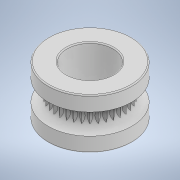
# Autodesk Inventor part: ToothedLoadedWheel_10mm
Saved by Autodesk Inventor 2021 (Build 250183000, 183)
## iProperties
Created: 2021-07-08
Part Number: ToothedLoadedWheel_10mm
Material: Generic
Document SubType Name: Modeling
Designer: zmac845
Density: 1 g/cm^3
Appearance: Default
Author: zmac845
Autodesk Inventor part; units mm, degrees
ref_plane "YZ Plane" through (0, 0, 0) normal (1, 0, 0) x (0, 1, 0)
ref_plane "XZ Plane" through (0, 0, 0) normal (0, 1, 0) x (-1, 0, 0)
ref_plane "XY Plane" through (0, 0, 0) normal (0, 0, 1) x (1, 0, 0)
sketch "Sketch1" plane through (0, 0, 0) normal (0, 0, 1) x (1, 0, 0)
  line L0 (0, 0) -> (20, 0)
  line L1 (20, 0) -> (20, 12)
  line L2 (20, 12) -> (0, 12)
  line L3 (0, 12) -> (0, 0)
  line L4 (0, 0) -> (11, 0)
  line L5 (11, 0) -> (11, 12)
  line L6 (11, 12) -> (0, 12)
  line L7 (0, 12) -> (0, 0)
  line L8 (20, 12) -> (20, 12)
  arc A0 (15, 12) -> (23.1054, 8.0813) centre (20, 12) ccw
  point P0 (20, 7)
  dimension "d0" = 20
  dimension "d1" = 12
  dimension "d2" = 11
  dimension "d3" = 0
  dimension "d4" = 5
  constraints: 18 end point, 4 parallel, 3 perpendicular, 2 horizontal, 2 point on circle, 2 point on line, 1 centre point, 1 coincident
  measures "d0" distance of L2.end L1.end
  measures "d1" distance of L1.end L0.end
  measures "d2" distance of L6.end L5.end
  measures "d3" distance of L1.end L8.end
  measures "d4" radius of A0
revolve "Revolution1" add sketch "Sketch1" angle 360 about axis through (0, 12, 0) along (0, -1, 0) contours L5 L2 A0 L1 L0
mirror "Mirror1" about plane through (15, 12, 0) normal (0, 1, 0) of "Revolution1"
fillet "Fillet1" radius 0.5 4 edges at (-20, 0, 0) (-11, 0, 0) (-20, 24, 0) (-11, 24, 0)
sketch "Sketch2" plane through (0, 24, 0) normal (0, 1, 0) x (1, 0, 0)
  circle A0 centre (0, 0) radius 15
  line L0 (-11.25, 11.25) -> (11.25, 11.25)
  line L1 (11.25, 11.25) -> (11.25, -11.25)
  line L2 (11.25, -11.25) -> (-11.25, -11.25)
  line L3 (-11.25, -11.25) -> (-11.25, 11.25)
  point P0 (-11.25, 9.9216)
  point P1 (-9.9216, 11.25)
  dimension "d7" = 30
  dimension "d8" = 22.5
  dimension "d9" = 22.5
  dimension "d10" = 11.25
  dimension "d11" = 11.25
  constraints: 8 end point, 2 parallel, 1 centre point, 1 coincident, 1 horizontal, 1 perpendicular
  measures "d7" diameter of A0
  measures "d8" distance of L0.start L0.end
  measures "d9" distance of L2.end L0.start
  measures "d10" distance from line of point (0, 0) L0
  measures "d11" distance from line of L1 point (0, 0)
extrude "Extrusion1" add sketch "Sketch2" against normal blind 24 contours A0 L3 L0
pattern_circular "Circular Pattern1" count 36 over 360 about axis through (0, 20.5, 0) along (0, -1, 0) of "Extrusion1"
body "Solid1"
